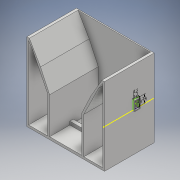
# Autodesk Inventor part: qzawsxedcfvgbhnjmk,l.
Saved by Autodesk Inventor 2020.3 (Build 243373000, 373)
## iProperties
Part Number: qzawsxedcfvgbhnjmk,l.
Material: Типовые
Document SubType Name: Modeling
Designer: ahmad
Density: 1 g/cm^3
Appearance: По умолчанию
Author: ahmad
Autodesk Inventor part; units mm, degrees
ref_plane "YZ Plane" through (0, 0, 0) normal (1, 0, 0) x (0, 1, 0)
ref_plane "XZ Plane" through (0, 0, 0) normal (0, 1, 0) x (-1, 0, 0)
ref_plane "XY Plane" through (0, 0, 0) normal (0, 0, 1) x (1, 0, 0)
sketch "Эскиз1" plane through (0, 0, 0) normal (0, 1, 0) x (-1, 0, 0)
  line L0 (-115, -115) -> (115, -115)
  line L1 (115, -115) -> (115, 115)
  line L2 (-115, 115) -> (-115, -115)
  line L3 (-115, -115) -> (115, 115) construction
  line L4 (115, -115) -> (-115, 115) construction
  line L5 (-107.5, -107.5) -> (107.5, -107.5)
  line L6 (107.5, -107.5) -> (107.5, 107.5)
  line L7 (-107.5, 107.5) -> (-107.5, -107.5)
  line L8 (-107.5, -107.5) -> (107.5, 107.5) construction
  line L9 (107.5, -107.5) -> (-107.5, 107.5) construction
  line L10 (107.5, 107.5) -> (107.5, 115)
  line L11 (-107.5, 107.5) -> (-107.5, 115)
  line L12 (115, 115) -> (107.5, 115)
  line L13 (-107.5, 115) -> (-115, 115)
  line L14 (107.5, 115) -> (74.5, 57.8423)
  line L15 (107.5, 115) -> (173.5, 115) construction
  line L16 (74.5, 57.8423) -> (47.5277, 0)
  line L17 (74.5, 57.8423) -> (138.3219, 57.8423) construction
  line L18 (47.5277, 0) -> (47.5277, -107.5)
  line L19 (-107.5, 115) -> (-74.5, 57.8423)
  line L20 (-107.5, 115) -> (-41.5, 115) construction
  line L21 (-74.5, 57.8423) -> (-47.5277, 0)
  line L22 (-74.5, 57.8423) -> (-10.6781, 57.8423) construction
  line L23 (-47.5277, 0) -> (-47.5277, -107.5)
  point P0 (0, 0)
  dimension "d0" = 230
  dimension "d1" = 230
  dimension "d4" = 66
  dimension "d5" = 120
  dimension "d6" = 115
  dimension "d7" = 66
  dimension "d8" = 60
  dimension "d9" = 65
  constraints: 48 end point, 6 horizontal, 5 perpendicular, 4 equal length, 4 midpoint, 4 parallel, 2 point on line, 2 vertical
  measures "d0" distance of L2.start L1.end
  measures "d1" distance of L1.end L0.end
  measures "d4" distance of L10.end L14.end
  measures "d5" angle of L14 L15
  measures "d6" angle of L16 L17
  measures "d7" distance of L11.end L19.end
  measures "d8" angle of L19 L20
  measures "d9" angle of L21 L22
extrude "Выдавливание1" add sketch "Эскиз1" along normal blind 150
sketch "Эскиз2" plane through (0, 150, 0) normal (0, 1, 0) x (1, 0, 0)
  line L0 (97.5879, -89.6233) -> (53.6439, -0.306)
  line L1 (53.6439, -0.306) -> (53.6439, 108.3759)
  line L2 (53.6439, 108.3759) -> (109.6776, 108.3759)
  line L3 (109.6776, 108.3759) -> (109.6776, -107.4647)
  line L4 (109.6776, -107.4647) -> (97.5879, -89.6233)
  line L5 (0, -179.4064) -> (0, 240.0482)
  line L6 (-97.5879, -89.6233) -> (-53.6439, -0.306)
  line L7 (-53.6439, -0.306) -> (-53.6439, 108.3759)
  line L8 (-53.6439, 108.3759) -> (-109.6776, 108.3759)
  line L9 (-109.6776, 108.3759) -> (-109.6776, -107.4647)
  line L10 (-109.6776, -107.4647) -> (-97.5879, -89.6233)
  point P0 (0, 0)
  constraints: 22 end point, 5 symmetric about line, 3 vertical, 1 perpendicular
extrude "Выдавливание2" cut sketch "Эскиз2" against normal blind 135161
sketch "Эскиз3" plane through (0, 150, 0) normal (0, 1, 0) x (1, 0, 0)
  line L0 (-107.5, -115) -> (-115, -115) projected
  line L1 (115, 115) -> (-115, 115)
  line L2 (-115, 115) -> (-115, -115)
  line L3 (-115, -115) -> (115, -115)
  line L4 (115, -115) -> (115, 115)
  line L5 (115, 115) -> (-115, -115) construction
  line L6 (-115, 115) -> (115, -115) construction
  point P0 (0, 0)
  constraints: 12 end point, 2 midpoint, 2 parallel, 1 horizontal, 1 perpendicular
extrude "Выдавливание3" add sketch "Эскиз3" against normal blind 3
sketch "Эскиз4" plane through (0, 0, 0) normal (0, -1, 0) x (1, 0, 0)
  line L0 (-115, -115) -> (115, -115) projected
  line L1 (115, 115) -> (-115, 115)
  line L2 (-115, 115) -> (-115, -115)
  line L3 (-115, -115) -> (115, -115)
  line L4 (115, -115) -> (115, 115)
  line L5 (115, 115) -> (-115, -115) construction
  line L6 (-115, 115) -> (115, -115) construction
  point P0 (0, 0)
  dimension "d16" = 230
  dimension "d17" = 230
  constraints: 12 end point, 2 midpoint, 2 parallel, 1 horizontal, 1 perpendicular
  measures "d16" distance of L3.end L0.start
  measures "d17" distance of L0.start L1.end
extrude "Выдавливание4" cut sketch "Эскиз4" against normal blind 3
sketch "Эскиз5" plane through (-47.5277, 147, -107.5) normal (0, 0, 1) x (1, 0, 0)
  line L0 (95.0554, -144) -> (95.0554, 0) projected
  line L1 (-0.0319, -84.1415) -> (95.0554, -84.1415)
  line L2 (95.0554, -84.1415) -> (95.0554, -74.1415)
  line L3 (95.0554, -74.1415) -> (-0.0319, -74.1415)
  line L4 (-0.0319, -74.1415) -> (-0.0319, -84.1415)
  point P0 (47.5277, -147)
  dimension "d20" = 10
  constraints: 8 end point, 2 parallel, 1 horizontal, 1 perpendicular, 1 point on line
  measures "d20" distance of L2.end L1.end
extrude "Выдавливание5" add sketch "Эскиз5" along normal blind 10
sketch "Эскиз6" plane through (53.6439, 147, 0.306) normal (1, 0, 0) x (0, 0, -1)
  line L0 (107.806, -74.1415) -> (97.806, -74.1415) projected
  line L1 (97.806, -74.1415) -> (97.806, -84.1415) projected
  line L2 (97.806, -84.1415) -> (107.806, -84.1415) projected
  line L3 (107.806, -144) -> (107.806, -84.1415) projected
  line L4 (107.806, -144) -> (0.306, -144) projected
  line L5 (0.306, -144) -> (0.306, 0) projected
  line L6 (0.306, 0) -> (107.806, 0) projected
  line L7 (107.806, -74.1415) -> (107.806, 0) projected
  circle A0 centre (102.806, -79.1415) radius 3.5
  point P0 (0.306, -147)
  dimension "d23" = 7
  constraints: 1 centre point
  measures "d23" diameter of A0
extrude "Выдавливание6" cut sketch "Эскиз6" against normal blind 113.25 contours A0
sketch "Эскиз7" plane through (115, 150, 115) normal (1, 0, 0) x (0, 0, -1)
  line L0 (114.694, -3) -> (114.694, -147) projected
  line L1 (114.694, -60.802) -> (90.694, -60.802)
  line L2 (90.694, -60.802) -> (90.694, -48.802)
  line L3 (90.694, -48.802) -> (114.694, -48.802)
  line L4 (114.694, -48.802) -> (114.694, -60.802)
  line L5 (116.694, -62.802) -> (88.694, -62.802)
  line L6 (88.694, -62.802) -> (88.694, -46.802)
  line L7 (88.694, -46.802) -> (116.694, -46.802)
  line L8 (116.694, -46.802) -> (116.694, -62.802)
  line L9 (116.694, -62.802) -> (88.694, -46.802) construction
  line L10 (88.694, -62.802) -> (116.694, -46.802) construction
  point P0 (115, -150)
  point P1 (102.694, -54.802)
  point P2 (114.694, -48.802)
  dimension "d26" = 24
  dimension "d27" = 12
  dimension "d28" = 28
  dimension "d29" = 16
  constraints: 20 end point, 4 parallel, 2 horizontal, 2 midpoint, 2 perpendicular, 1 point on line
  measures "d26" distance of L2.end L3.end
  measures "d27" distance of L1.end L2.end
  measures "d28" distance of L6.end L7.end
  measures "d29" distance of L5.end L6.end
extrude "Выдавливание7" add sketch "Эскиз7" along normal blind 5 contours L0 L7 L8 L5 | L3 L2 L1 L0 L5 L6 L7
extrude "Выдавливание8" cut sketch "Эскиз7" against normal blind 44.75 contours L0 L1 L2 L3
pattern_linear "Прямоуг.массив1" count 2 spacing 235 along (-1, 0, 0) of "Выдавливание7"
sketch "Эскиз8" plane through (-115, 89.198, 0.306) normal (-1, 0, 0) x (0, 0, 1)
  line L0 (24, 12) -> (24, 0) projected
  line L1 (24, 12) -> (0, 12) projected
  line L2 (24, 0) -> (0, 0)
  line L3 (0, 0) -> (0, 12)
  line L4 (0, 12) -> (24, 12)
  line L5 (24, 12) -> (24, 0)
  point P0 (-0.306, -89.198)
  constraints: 8 end point, 2 parallel, 1 horizontal, 1 perpendicular
extrude "Выдавливание9" cut sketch "Эскиз8" against normal blind 18
